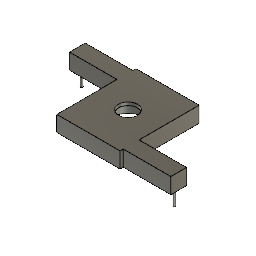
Rack n Rod Connector (Autodesk Fusion 360 design; units mm, degrees)
Autodesk Fusion 360 part; units mm, degrees
sketch "Top" plane through (0, 0, 0) normal (0, 0, 1) x (1, 0, 0)
  line L0 (0, 0) -> (40, 0)
  line L1 (40, 0) -> (40, 50)
  line L2 (40, 50) -> (0, 50)
  line L3 (0, 50) -> (0, 0)
  circle A0 centre (20, 25) radius 11.2
  circle A1 centre (20, 25) radius 6
  dimension "d6" = 40
  dimension "d7" = 50
  dimension "d11" = 22.4
  dimension "d12" = 25
  dimension "d13" = 20
  dimension "d27" = 12
  constraint horizontal L0
  constraint vertical L1
  constraint horizontal L2
  constraint vertical L3
  constraint coincident L0.start L3.end
  constraint concentric A0 A1
  measures "d6" distance of L0.start L0.end
  measures "d7" distance of L0.start L2.end
  measures "d11" diameter of A0
  measures "d12" distance of L2 A0.centre
  measures "d13" distance of L1 A0.centre
  measures "d27" diameter of A1
extrude "Extrude1" add sketch "Top" along normal blind 10 contours L0 L1 L2 L3 | A0 | A1
extrude "Extrude2" cut sketch "Top" along normal blind 8 contours A0 | A1
extrude "Extrude5" cut sketch "Top" along normal blind 110 contours A1
sketch "Sketch5" plane through (0, 0, 0) normal (-1, 0, 0) x (0, -1, 0)
  line L0 (-50, 0) -> (0, 0)
  line L1 (0, 0) -> (0, 10)
  line L2 (0, 10) -> (-50, 10)
  line L3 (-50, 10) -> (-50, 0)
  line L4 (-48, 10) -> (-38, 10)
  line L5 (-38, 10) -> (-38, 0)
  line L6 (-38, 0) -> (-48, 0)
  line L7 (-48, 0) -> (-48, 10)
  dimension "d50" = 10
  dimension "d51" = 10
  dimension "d52" = 2
  constraint horizontal L4
  constraint vertical L5
  constraint horizontal L6
  constraint vertical L7
  constraint coincident L2 L4.start
  measures "d50" distance of L4.start L4.end
  measures "d51" distance of L4.start L6.end
  measures "d52" distance of L3 L7
extrude "Extrude8" add sketch "Sketch5" along normal blind 30 contours L0 L2 L4 L5 L6 L7
sketch "Sketch8" plane through (40, 0, 0) normal (1, 0, 0) x (0, 1, 0)
  line L0 (0, 0) -> (50, 0)
  line L1 (50, 0) -> (50, 10)
  line L2 (50, 10) -> (0, 10)
  line L3 (0, 10) -> (0, 0)
  line L4 (2, 10) -> (12, 10)
  line L5 (12, 10) -> (12, 0)
  line L6 (12, 0) -> (2, 0)
  line L7 (2, 0) -> (2, 10)
  dimension "d72" = 10
  dimension "d73" = 10
  dimension "d74" = 2
  constraint horizontal L4
  constraint vertical L5
  constraint horizontal L6
  constraint vertical L7
  constraint coincident L2 L4.start
  measures "d72" distance of L4.start L6.end
  measures "d73" distance of L4.start L4.end
  measures "d74" distance of L3 L7
extrude "Extrude11" add sketch "Sketch8" along normal blind 30 contours L0 L2 L4 L5 L6 L7
sketch "Sketch9" plane through (0, 0, 0) normal (0, 0, -1) x (1, 0, 0)
  circle A0 centre (20, -25) radius 11.2
  line L0 (0, -48) -> (0, -50)
  line L1 (0, -50) -> (40, -50)
  line L2 (40, -50) -> (40, -12)
  line L3 (40, -12) -> (70, -12)
  line L4 (70, -12) -> (70, -2)
  line L5 (70, -2) -> (40, -2)
  line L6 (40, -2) -> (40, 0)
  line L7 (40, 0) -> (0, 0)
  line L8 (0, 0) -> (0, -38)
  line L9 (0, -38) -> (-30, -38)
  line L10 (-30, -38) -> (-30, -48)
  line L11 (-30, -48) -> (0, -48)
  circle A1 centre (-27.2, -43) radius 0.8
  circle A2 centre (67.2, -7) radius 0.8
  dimension "d81" = 1.6
  dimension "d82" = 1.6
  dimension "d83" = 2.8
  dimension "d84" = 5
  dimension "d85" = 2.8
  dimension "d86" = 5
  measures "d81" diameter of A1
  measures "d82" diameter of A2
  measures "d83" distance of L10 A1.centre
  measures "d84" distance of L9 A1.centre
  measures "d85" distance of L4 A2.centre
  measures "d86" distance of L5 A2.centre
extrude "Extrude12" add sketch "Sketch9" along normal blind 10 contours A1 | A2
equation "length = 50 mm"
equation "width = 40 mm"
equation "thickness = 10 mm"
equation "extra = 100 mm"
equation "fit_gap = 0.2 mm"
equation "d6 = width"
equation "d7 = length"
equation "d8 = thickness"
equation "bearing_outer_radius = 11.1 mm"
equation "d11 = ( bearing_outer_radius * 2 ) + fit_gap"
equation "d12 = length / 2"
equation "d13 = width / 2"
equation "d14 = thickness - 2 mm"
equation "bearing_inner_radius = ( 8 mm + 4 mm ) / 2"
equation "d27 = bearing_inner_radius * 2"
equation "d28 = thickness + extra"
equation "rack_rock_bracket_length = 30 mm"
equation "rack_rock_bracket_width = 10 mm"
equation "rack_rock_bracket_big_distance = 2 mm"
equation "d50 = rack_rock_bracket_width"
equation "d51 = rack_rock_bracket_width"
equation "d52 = rack_rock_bracket_big_distance"
equation "d53 = rack_rock_bracket_length"
equation "d72 = rack_rock_bracket_width"
equation "d73 = rack_rock_bracket_width"
equation "d74 = rack_rock_bracket_big_distance"
equation "d75 = rack_rock_bracket_length"
equation "bearing_dowel_radius = 0.8 mm"
equation "bearing_dowel_length = 10 mm"
equation "bearing_dowel_big_distance = 2 mm + bearing_dowel_radius"
equation "bearing_dowel_small_distance = rack_rock_bracket_width / 2"
equation "d81 = bearing_dowel_radius * 2"
equation "d82 = bearing_dowel_radius * 2"
equation "d83 = bearing_dowel_big_distance"
equation "d84 = bearing_dowel_small_distance"
equation "d85 = bearing_dowel_big_distance"
equation "d86 = bearing_dowel_small_distance"
equation "d87 = bearing_dowel_length"
